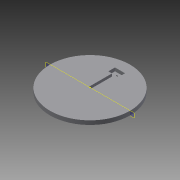
# Autodesk Inventor part: base_botella
Saved by Autodesk Inventor 2015 SP1 (Build 190203100, 203)
## iProperties
Created: 2015-07-05
Part Number: base_botella
Material: Genérico
Document SubType Name: Modeling
Designer: Javier
Density: 1 g/cm^3
Appearance: Valor por defecto
Author: Javier
Autodesk Inventor part; units mm, degrees
ref_plane "YZ Plane" through (0, 0, 0) normal (1, 0, 0) x (0, 1, 0)
ref_plane "XY Plane" through (0, 0, 0) normal (0, 0, 1) x (1, 0, 0)
sketch "Boceto1" plane through (0, 0, 0) normal (0, 0, 1) x (1, 0, 0)
  circle A0 centre (0, 0) radius 60
  dimension "d0" = 120
  constraints: 1 centre point, 1 coincident
  measures "d0" diameter of A0
extrude "Extrusión1" add sketch "Boceto1" along normal blind 6
sketch "Boceto2" plane through (0, 0, 6) normal (0, 0, 1) x (1, 0, 0)
  point P0 (0, 0)
sketch "Boceto3" plane through (0, 0, 6) normal (0, 0, 1) x (1, 0, 0)
  line L0 (-7.5, 35) -> (7.5, 35)
  line L1 (7.5, 35) -> (7.5, 45)
  line L2 (7.5, 45) -> (-7.5, 45)
  line L3 (-7.5, 45) -> (-7.5, 35)
  line L4 (-7.5, 35) -> (7.5, 45) construction
  line L5 (7.5, 35) -> (-7.5, 45) construction
  line L6 (0, 0) -> (0, 35)
  point P0 (0, 40)
  dimension "d3" = 15
  dimension "d4" = 10
  dimension "d14" = 35
  constraints: 14 end point, 3 midpoint, 2 parallel, 1 horizontal, 1 perpendicular, 1 point on line, 1 vertical
  measures "d3" distance of L2.end L1.end
  measures "d4" distance of L1.end L0.end
  measures "d14" distance of L6.start L6.end
extrude "Extrusión2" cut sketch "Boceto3" against normal blind 5
sketch "Boceto4" plane through (0, 0, 1) normal (0, 0, 1) x (1, 0, 0)
  circle A0 centre (0, 25) radius 1.5
  line L0 (7.5, 35) -> (-7.5, 35) projected
  line L1 (7.5, 45) -> (7.5, 35) projected
  line L2 (-7.5, 45) -> (7.5, 45) projected
  line L3 (-7.5, 35) -> (-7.5, 45) projected
  circle A1 centre (0, 40) radius 1.5
  point P0 (0, 0)
  dimension "d7" = 3
  dimension "d17" = 3
  constraints: 2 centre point, 1 coincident
  measures "d7" diameter of A0
  measures "d17" diameter of A1
extrude "Extrusión3" cut sketch "Boceto4" against normal blind 5 contours A1
sketch "Boceto5" plane through (0, 0, 6) normal (0, 0, 1) x (1, 0, 0)
  line L0 (0, 0) -> (-2, 0)
  line L1 (-7.5, 35) -> (-7.5, 45) projected
  line L2 (7.5, 35) -> (-7.5, 35) projected
  line L3 (-7.5, 45) -> (7.5, 45) projected
  line L4 (7.5, 45) -> (7.5, 35) projected
  line L5 (-2, 0) -> (-2, 35)
  line L6 (7.5, 35) -> (-7.5, 35) projected
  line L7 (0, 0) -> (2, 0)
  line L8 (2, 0) -> (2, 35)
  dimension "d15" = 2
  dimension "d16" = 2
  constraints: 8 end point, 3 perpendicular, 2 point on line, 1 horizontal
  measures "d15" distance of L0.start L0.end
  measures "d16" distance of L0.start L7.end
extrude "Extrusión4" cut sketch "Boceto5" against normal up to surface (5 mm away) contours L0 L5 L2 L8 L7
